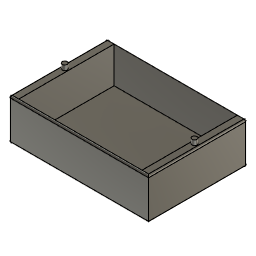
Boitier_Arduino_2 v5 (Autodesk Fusion 360 design; units mm, degrees)
Autodesk Fusion 360 part; units mm, degrees
sketch "Esquisse1" plane through (0, 0, 0) normal (0, 0, 1) x (1, 0, 0)
  line L0 (0, 0) -> (85, 0)
  line L1 (85, 0) -> (85, 60)
  line L2 (85, 60) -> (0, 60)
  line L3 (0, 60) -> (0, 0)
  dimension "d3" = 85
  dimension "d4" = 60
  constraint horizontal L0
  constraint vertical L1
  constraint horizontal L2
  constraint vertical L3
  constraint coincident L0.start L3.end
  measures "d3" distance of L1.end L2.end
  measures "d4" distance of L0.end L1.end
extrude "Extrusion1" add sketch "Esquisse1" along normal blind 25
fillet "Congé1" radius 1 11 edges at (0, 30, 25) (0, 30, 0) (42.5, 0, 0) (85, 30, 25) (42.5, 0, 25) (42.5, 60, 25) (85, 30, 0) (42.5, 60, 0) (85, 60, 12.5) (0, 0, 12.5) (0, 60, 12.5)
sketch "Esquisse2" plane through (0, 0, 25) normal (0, 0, 1) x (-1, 0, 0)
  line L0 (-84, -1) -> (-84, -59)
  line L1 (-84, -59) -> (-1, -59)
  line L2 (-1, -59) -> (-1, -1)
  line L3 (-1, -1) -> (-84, -1)
  line L4 (-84, -1) -> (-80, -1)
  line L5 (-80, -1) -> (-80, -59)
  line L6 (-80, -59) -> (-84, -59)
  line L7 (-84, -59) -> (-84, -1)
  line L8 (-1, -1) -> (-5, -1)
  line L9 (-5, -1) -> (-5, -59)
  line L10 (-5, -59) -> (-1, -59)
  line L11 (-1, -59) -> (-1, -1)
  dimension "d11" = 4
  dimension "d12" = 4
  constraint horizontal L4
  constraint vertical L5
  constraint horizontal L6
  constraint vertical L7
  constraint coincident L1 L5.end
  constraint coincident L0.start L3.end
  constraint horizontal L8
  constraint vertical L9
  constraint horizontal L10
  constraint vertical L11
  constraint coincident L1 L9.end
  constraint coincident L2.end L3.start
  measures "d11" distance of L5.end L0.end
  measures "d12" distance of L9.end L1.end
extrude "Extrusion2" cut sketch "Esquisse2" against normal blind 22 contours L1 L3 L5 L9
sketch "Esquisse3" plane through (0, 0, 25) normal (0, 0, 1) x (-1, 0, 0)
  line L0 (-80, -59) -> (-80, -1)
  line L1 (-80, -1) -> (-84, -1)
  line L2 (-84, -1) -> (-84, -59)
  line L3 (-84, -59) -> (-80, -59)
  circle A0 centre (-82, -31) radius 1.5
  line L4 (-82, -31) -> (16.3058, -31) construction
  circle A1 centre (-3, -31) radius 1.5
  line L5 (-5, -1) -> (-5, -59) construction
  line L6 (-80, -1) -> (-5, -1)
  dimension "d15" = 2
  dimension "d17" = 3
  dimension "d18" = 2
  dimension "d36" = 30
  constraint coincident A0.centre L4.start
  constraint perpendicular L2 L4
  constraint coincident L4 A1.centre
  constraint equal A0 A1
  measures "d15" distance of L0 A0.centre
  measures "d17" diameter of A0
  measures "d18" distance of A1.centre L5
  measures "d36" distance of L4 L6
extrude "Extrusion3" add sketch "Esquisse3" along normal blind 3 contours A0 | A1
sketch "Esquisse4" plane through (85, 0, 0) normal (1, 0, 0) x (0, 1, 0)
  line L0 (59, 24) -> (0, 24)
  line L1 (0, 24) -> (0, 1)
  line L2 (0, 1) -> (59, 1)
  line L3 (59, 1) -> (59, 24)
  line L4 (10.5, 8.5) -> (20.5, 8.5)
  line L5 (20.5, 8.5) -> (20.5, 4)
  line L6 (20.5, 4) -> (10.5, 4)
  line L7 (10.5, 4) -> (10.5, 8.5)
  line L8 (44, 17) -> (55, 17)
  line L9 (55, 17) -> (55, 4)
  line L10 (55, 4) -> (44, 4)
  line L11 (44, 4) -> (44, 17)
  dimension "d22" = 10.5
  dimension "d23" = 10
  dimension "d24" = 4.5
  dimension "d25" = 3
  dimension "d27" = 13
  dimension "d28" = 11
  dimension "d29" = 4
  constraint horizontal L4
  constraint vertical L5
  constraint horizontal L6
  constraint vertical L7
  constraint horizontal L8
  constraint vertical L9
  constraint horizontal L10
  constraint vertical L11
  constraint collinear L6 L10
  measures "d22" distance of L1 L7
  measures "d23" distance of L4.start L4.end
  measures "d24" distance of L4.end L5.end
  measures "d25" distance of L2 L6
  measures "d27" distance of L8.end L9.end
  measures "d28" distance of L8.start L8.end
  measures "d29" distance of L3 L9
extrude "Extrusion4" [suppressed]
fillet "Congé2" [suppressed]
copy_body "Corps->Comp1" [suppressed] in component "Boitier"
equation "longueur = 85 mm"
equation "largeur = 60 mm"
equation "d3 = longueur"
equation "d4 = largeur"
equation "d5 = volume"
equation "volume = 25 mm"
equation "longueur_support = 4 mm"
equation "d11 = longueur_support"
equation "d12 = longueur_support"
equation "d15 = longueur_support / 2"
equation "rayon_accroche = 3 mm"
equation "d17 = rayon_accroche"
equation "d18 = longueur_support / 2"
equation "d19 = extrusion_support"
equation "extrusion_support = 3 mm"
equation "d23 = longueur_cable_usb"
equation "d24 = hauteur_cable_usb"
equation "d27 = hauteur_prise_jack"
equation "d28 = longueur_prise_jack"
equation "d36 = largeur / 2"
equation "longueur_prise_jack = 11 mm"
equation "hauteur_prise_jack = 13 mm"
equation "longueur_cable_usb = 10 mm"
equation "hauteur_cable_usb = 4.5 mm"
